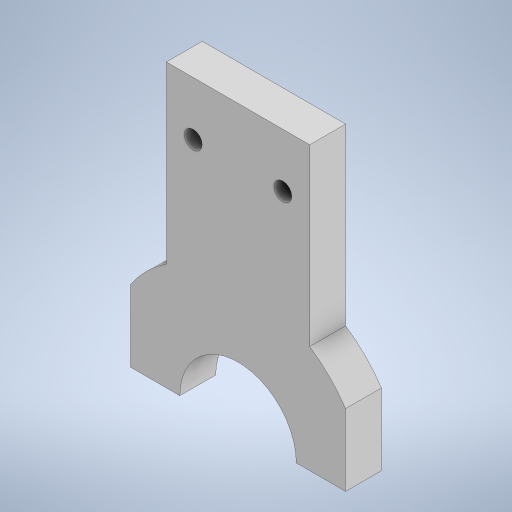
# Autodesk Inventor part: Frame Middle
Saved by Autodesk Inventor 2023 (Build 270158000, 158)
## iProperties
Created: 2022-10-29
Part Number: Frame Middle
Material: Generic
Document SubType Name: Modeling
Designer: tommy
Density: 1 g/cm^3
Appearance: Default
Author: tommy
Autodesk Inventor part; units mm, degrees
ref_plane "YZ Plane" through (0, 0, 0) normal (1, 0, 0) x (0, 1, 0)
ref_plane "XZ Plane" through (0, 0, 0) normal (0, 1, 0) x (-1, 0, 0)
ref_plane "XY Plane" through (0, 0, 0) normal (0, 0, 1) x (1, 0, 0)
sketch "Sketch1" plane through (0, 0, 0) normal (0, 0, 1) x (1, 0, 0)
  circle A0 centre (25.4426, 130.4898) radius 3.175
  circle A1 centre (57.1926, 130.4898) radius 3.175
  line L0 (55.6051, 149.5398) -> (27.0301, 149.5398)
  line L1 (41.3176, 149.5398) -> (41.3176, 49.5146)
  arc A2 (61.9551, 49.5146) -> (20.6801, 49.5146) centre (41.3176, 49.5146) ccw
  line L2 (66.7176, 87.6146) -> (66.7176, 149.5398)
  line L3 (15.9176, 87.6146) -> (15.9176, 149.5398)
  line L4 (79.4176, 49.5146) -> (79.4176, 72.4098)
  line L5 (3.2176, 49.5146) -> (3.2176, 72.4098)
  line L6 (66.7176, 149.5398) -> (15.9176, 149.5398)
  line L7 (3.2176, 49.5146) -> (79.4176, 49.5146)
  line L8 (79.4176, 49.5146) -> (79.4176, 74.9146)
  line L9 (3.2176, 49.5146) -> (3.2176, 74.9146)
  arc A3 (15.9176, 87.6146) -> (3.2176, 74.9146) centre (41.3176, 49.5146) ccw
  arc A4 (79.4176, 74.9146) -> (66.7176, 87.6146) centre (41.3176, 49.5146) ccw
  point P0 (27.0301, 149.5398)
  dimension "d2" = 6.35
  dimension "d3" = 6.35
  dimension "d6" = 100.0252
  dimension "d7" = 41.275
  dimension "d18" = 19.05
  dimension "d19" = 19.05
  dimension "d20" = 25.4
  dimension "d21" = 25.4
  constraints: 20 end point, 6 point on circle, 5 centre point, 3 point on line, 2 midpoint, 2 vertical, 1 coincident
  measures "d2" diameter of A0
  measures "d3" diameter of A1
  measures "d6" distance of L1.start L1.end
  measures "d7" diameter of A2
  measures "d18" distance from line of L6 A1.centre
  measures "d19" vertical distance of L0.end A0.centre
  measures "d20" distance of L4.start L8.end
  measures "d21" distance of L5.start L9.end
extrude "Extrusion3" add sketch "Sketch1" along normal blind 12.7 contours L6 L2 A4 L8 L4 L7 A2 L1 L0 | L1 A2 L7 L5 L9 A3 L3 L6 L0
body "Solid3"
